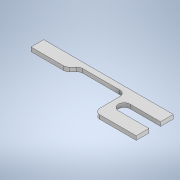
# Autodesk Inventor part: harveyLabWideHeadplate_1p4in
Saved by Autodesk Inventor 2022.1 (Build 261234000, 234)
## iProperties
Created: 2022-07-07
Part Number: harveyLabWideHeadplate_1p4in
Material: Generic
Document SubType Name: Modeling
Designer: Noah
Density: 1 g/cm^3
Appearance: Default
Author: Noah
Autodesk Inventor part; units mm, degrees
ref_plane "YZ Plane" through (0, 0, 0) normal (1, 0, 0) x (0, 1, 0)
ref_plane "XZ Plane" through (0, 0, 0) normal (0, 1, 0) x (-1, 0, 0)
ref_plane "XY Plane" through (0, 0, 0) normal (0, 0, 1) x (1, 0, 0)
sketch "Sketch1" plane through (0, 0, 0) normal (0, 1, 0) x (-1, 0, 0)
  line L0 (3.3655, -3.556) -> (-3.3655, -3.556)
  line L1 (-12.7, 1.5875) -> (-9.398, 1.5875)
  line L2 (-9.398, -1.5875) -> (-12.7, -1.5875)
  line L3 (-12.7, -5.08) -> (12.7, -5.08)
  line L4 (12.7, -1.5875) -> (8.8491, -1.5875)
  line L5 (-12.7, -5.08) -> (-17.78, -5.08)
  line L6 (-17.78, -5.08) -> (-17.78, -1.5875)
  line L7 (-17.78, -1.5875) -> (-12.7, -1.5875)
  line L8 (-12.7, 1.5875) -> (-17.78, 1.5875)
  line L9 (-17.78, 1.5875) -> (-17.78, 5.08)
  line L10 (12.7, -5.08) -> (17.78, -5.08)
  line L11 (17.78, -5.08) -> (17.78, -1.5875)
  line L12 (17.78, -1.5875) -> (12.7, -1.5875)
  line L13 (12.7, -1.5875) -> (8.8491, -1.5875)
  line L14 (-8.128, 0) -> (-9.398, 0)
  line L15 (-3.3655, -3.556) -> (-4.6355, -3.556)
  line L16 (-6.223, -1.9685) -> (-6.223, 3.4925)
  arc A0 (-9.398, -1.5875) -> (-9.398, 1.5875) centre (-9.398, 0) ccw
  line L17 (-17.78, 5.08) -> (-7.8105, 5.08)
  line L18 (5.5654, -3.556) -> (3.3655, -3.556)
  line L19 (6.688, -3.091) -> (7.7265, -2.0525)
  line L20 (6.223, -3.556) -> (14.5183, -3.556) construction
  arc A1 (-6.223, -1.9685) -> (-4.6355, -3.556) centre (-4.6355, -1.9685) ccw
  arc A2 (-6.223, 3.4925) -> (-7.8105, 5.08) centre (-7.8105, 3.4925) ccw
  arc A3 (5.5654, -3.556) -> (6.688, -3.091) centre (5.5654, -1.9685) ccw
  arc A4 (8.8491, -1.5875) -> (7.7265, -2.0525) centre (8.8491, -3.175) ccw
  point P0 (0, 0)
  point P1 (-3.3655, -3.556)
  dimension "d0" = 5.08
  dimension "d1" = 5.08
  dimension "d3" = 1.27
  dimension "d6" = 45
  dimension "d7" = 1.5875
  constraints: 42 end point, 10 point on circle, 9 tangent, 7 horizontal, 5 centre point, 5 perpendicular, 3 equal radius, 2 point on line, 1 coincident, 1 collinear
  measures "d0" distance of L3.start L5.end
  measures "d1" distance of L10.start L10.end
  measures "d3" distance of L14.start L14.end
  measures "d6" angle of L20 L19
  measures "d7" radius of A1
extrude "Extrusion1" add sketch "Sketch1" along normal blind 1.1
body "Solid1"
